Autodesk Inventor part; units mm, degrees
(part 11 of 12)
  line L8976 (-20.439, 26.0176) -> (-20.439, 27.0176)
  line L8977 (-20.439, 27.0176) -> (-19.439, 27.0176)
  line L8978 (-19.439, 27.0176) -> (-19.439, 26.0176)
  line L8979 (-20.4042, 26.0176) -> (-21.4042, 26.0176)
  line L8980 (-21.4042, 26.0176) -> (-21.4042, 27.0176)
  line L8981 (-21.4042, 27.0176) -> (-20.4042, 27.0176)
  line L8982 (-20.4042, 27.0176) -> (-20.4042, 26.0176)
  line L8983 (-21.0011, 26.0176) -> (-22.0011, 26.0176)
  line L8984 (-22.0011, 26.0176) -> (-22.0011, 27.0176)
  line L8985 (-22.0011, 27.0176) -> (-21.0011, 27.0176)
  line L8986 (-21.0011, 27.0176) -> (-21.0011, 26.0176)
  line L8987 (-22.1187, 26.0176) -> (-23.1187, 26.0176)
  line L8988 (-23.1187, 26.0176) -> (-23.1187, 27.0176)
  line L8989 (-23.1187, 27.0176) -> (-22.1187, 27.0176)
  line L8990 (-22.1187, 27.0176) -> (-22.1187, 26.0176)
  line L8991 (-12.9747, 26.043) -> (-13.9747, 26.043)
  line L8992 (-13.9747, 26.043) -> (-13.9747, 27.043)
  line L8993 (-13.9747, 27.043) -> (-12.9747, 27.043)
  line L8994 (-12.9747, 27.043) -> (-12.9747, 26.043)
  line L8995 (-14.5415, 26.5303) -> (-14.5669, 26.5303)
  line L8996 (-14.5669, 26.5303) -> (-14.5669, 26.5557)
  line L8997 (-14.5669, 26.5557) -> (-14.5415, 26.5557)
  line L8998 (-14.5415, 26.5557) -> (-14.5415, 26.5303)
  line L8999 (-14.6257, 26.043) -> (-15.6257, 26.043)
  line L9000 (-15.6257, 26.043) -> (-15.6257, 27.043)
  line L9001 (-15.6257, 27.043) -> (-14.6257, 27.043)
  line L9002 (-14.6257, 27.043) -> (-14.6257, 26.043)
  line L9003 (-19.439, 26.043) -> (-20.439, 26.043)
  line L9004 (-20.439, 26.043) -> (-20.439, 27.043)
  line L9005 (-20.439, 27.043) -> (-19.439, 27.043)
  line L9006 (-19.439, 27.043) -> (-19.439, 26.043)
  line L9007 (-20.4169, 26.043) -> (-21.4169, 26.043)
  line L9008 (-21.4169, 26.043) -> (-21.4169, 27.043)
  line L9009 (-21.4169, 27.043) -> (-20.4169, 27.043)
  line L9010 (-20.4169, 27.043) -> (-20.4169, 26.043)
  line L9011 (-21.0011, 26.043) -> (-22.0011, 26.043)
  line L9012 (-22.0011, 26.043) -> (-22.0011, 27.043)
  line L9013 (-22.0011, 27.043) -> (-21.0011, 27.043)
  line L9014 (-21.0011, 27.043) -> (-21.0011, 26.043)
  line L9015 (-22.1314, 26.043) -> (-23.1314, 26.043)
  line L9016 (-23.1314, 26.043) -> (-23.1314, 27.043)
  line L9017 (-23.1314, 27.043) -> (-22.1314, 27.043)
  line L9018 (-22.1314, 27.043) -> (-22.1314, 26.043)
  line L9019 (-13.0128, 26.0684) -> (-14.0128, 26.0684)
  line L9020 (-14.0128, 26.0684) -> (-14.0128, 27.0684)
  line L9021 (-14.0128, 27.0684) -> (-13.0128, 27.0684)
  line L9022 (-13.0128, 27.0684) -> (-13.0128, 26.0684)
  line L9023 (-14.0415, 26.0684) -> (-15.0415, 26.0684)
  line L9024 (-15.0415, 26.0684) -> (-15.0415, 27.0684)
  line L9025 (-15.0415, 27.0684) -> (-14.0415, 27.0684)
  line L9026 (-14.0415, 27.0684) -> (-14.0415, 26.0684)
  line L9027 (-14.6257, 26.0684) -> (-15.6257, 26.0684)
  line L9028 (-15.6257, 26.0684) -> (-15.6257, 27.0684)
  line L9029 (-15.6257, 27.0684) -> (-14.6257, 27.0684)
  line L9030 (-14.6257, 27.0684) -> (-14.6257, 26.0684)
  line L9031 (-13.0382, 26.0938) -> (-14.0382, 26.0938)
  line L9032 (-14.0382, 26.0938) -> (-14.0382, 27.0938)
  line L9033 (-14.0382, 27.0938) -> (-13.0382, 27.0938)
  line L9034 (-13.0382, 27.0938) -> (-13.0382, 26.0938)
  line L9035 (-14.0161, 26.0938) -> (-15.0161, 26.0938)
  line L9036 (-15.0161, 26.0938) -> (-15.0161, 27.0938)
  line L9037 (-15.0161, 27.0938) -> (-14.0161, 27.0938)
  line L9038 (-14.0161, 27.0938) -> (-14.0161, 26.0938)
  line L9039 (-14.613, 26.0938) -> (-15.613, 26.0938)
  line L9040 (-15.613, 26.0938) -> (-15.613, 27.0938)
  line L9041 (-15.613, 27.0938) -> (-14.613, 27.0938)
  line L9042 (-14.613, 27.0938) -> (-14.613, 26.0938)
  line L9043 (-13.0382, 26.1192) -> (-14.0382, 26.1192)
  line L9044 (-14.0382, 26.1192) -> (-14.0382, 27.1192)
  line L9045 (-14.0382, 27.1192) -> (-13.0382, 27.1192)
  line L9046 (-13.0382, 27.1192) -> (-13.0382, 26.1192)
  line L9047 (-13.9907, 26.1192) -> (-14.9907, 26.1192)
  line L9048 (-14.9907, 26.1192) -> (-14.9907, 27.1192)
  line L9049 (-14.9907, 27.1192) -> (-13.9907, 27.1192)
  line L9050 (-13.9907, 27.1192) -> (-13.9907, 26.1192)
  line L9051 (-14.613, 26.1192) -> (-15.613, 26.1192)
  line L9052 (-15.613, 26.1192) -> (-15.613, 27.1192)
  line L9053 (-15.613, 27.1192) -> (-14.613, 27.1192)
  line L9054 (-14.613, 27.1192) -> (-14.613, 26.1192)
  line L9055 (-13.0255, 26.1446) -> (-14.0255, 26.1446)
  line L9056 (-14.0255, 26.1446) -> (-14.0255, 27.1446)
  line L9057 (-14.0255, 27.1446) -> (-13.0255, 27.1446)
  line L9058 (-13.0255, 27.1446) -> (-13.0255, 26.1446)
  line L9059 (-13.9653, 26.1446) -> (-14.9653, 26.1446)
  line L9060 (-14.9653, 26.1446) -> (-14.9653, 27.1446)
  line L9061 (-14.9653, 27.1446) -> (-13.9653, 27.1446)
  line L9062 (-13.9653, 27.1446) -> (-13.9653, 26.1446)
  line L9063 (-14.613, 26.1446) -> (-15.613, 26.1446)
  line L9064 (-15.613, 26.1446) -> (-15.613, 27.1446)
  line L9065 (-15.613, 27.1446) -> (-14.613, 27.1446)
  line L9066 (-14.613, 27.1446) -> (-14.613, 26.1446)
  line L9067 (-13.0128, 26.17) -> (-14.0128, 26.17)
  line L9068 (-14.0128, 26.17) -> (-14.0128, 27.17)
  line L9069 (-14.0128, 27.17) -> (-13.0128, 27.17)
  line L9070 (-13.0128, 27.17) -> (-13.0128, 26.17)
  line L9071 (-13.9526, 26.17) -> (-14.9526, 26.17)
  line L9072 (-14.9526, 26.17) -> (-14.9526, 27.17)
  line L9073 (-14.9526, 27.17) -> (-13.9526, 27.17)
  line L9074 (-13.9526, 27.17) -> (-13.9526, 26.17)
  line L9075 (-14.6003, 26.17) -> (-15.6003, 26.17)
  line L9076 (-15.6003, 26.17) -> (-15.6003, 27.17)
  line L9077 (-15.6003, 27.17) -> (-14.6003, 27.17)
  line L9078 (-14.6003, 27.17) -> (-14.6003, 26.17)
  line L9079 (-13.0001, 26.1954) -> (-14.0001, 26.1954)
  line L9080 (-14.0001, 26.1954) -> (-14.0001, 27.1954)
  line L9081 (-14.0001, 27.1954) -> (-13.0001, 27.1954)
  line L9082 (-13.0001, 27.1954) -> (-13.0001, 26.1954)
  line L9083 (-13.9272, 26.1954) -> (-14.9272, 26.1954)
  line L9084 (-14.9272, 26.1954) -> (-14.9272, 27.1954)
  line L9085 (-14.9272, 27.1954) -> (-13.9272, 27.1954)
  line L9086 (-13.9272, 27.1954) -> (-13.9272, 26.1954)
  line L9087 (-14.6003, 26.1954) -> (-15.6003, 26.1954)
  line L9088 (-15.6003, 26.1954) -> (-15.6003, 27.1954)
  line L9089 (-15.6003, 27.1954) -> (-14.6003, 27.1954)
  line L9090 (-14.6003, 27.1954) -> (-14.6003, 26.1954)
  line L9091 (-12.9747, 26.2208) -> (-13.9747, 26.2208)
  line L9092 (-13.9747, 26.2208) -> (-13.9747, 27.2208)
  line L9093 (-13.9747, 27.2208) -> (-12.9747, 27.2208)
  line L9094 (-12.9747, 27.2208) -> (-12.9747, 26.2208)
  line L9095 (-13.9018, 26.2208) -> (-14.9018, 26.2208)
  line L9096 (-14.9018, 26.2208) -> (-14.9018, 27.2208)
  line L9097 (-14.9018, 27.2208) -> (-13.9018, 27.2208)
  line L9098 (-13.9018, 27.2208) -> (-13.9018, 26.2208)
  line L9099 (-14.5876, 26.2208) -> (-15.5876, 26.2208)
  line L9100 (-15.5876, 26.2208) -> (-15.5876, 27.2208)
  line L9101 (-15.5876, 27.2208) -> (-14.5876, 27.2208)
  line L9102 (-14.5876, 27.2208) -> (-14.5876, 26.2208)
  line L9103 (-12.9747, 26.2462) -> (-13.9747, 26.2462)
  line L9104 (-13.9747, 26.2462) -> (-13.9747, 27.2462)
  line L9105 (-13.9747, 27.2462) -> (-12.9747, 27.2462)
  line L9106 (-12.9747, 27.2462) -> (-12.9747, 26.2462)
  line L9107 (-13.8891, 26.2462) -> (-14.8891, 26.2462)
  line L9108 (-14.8891, 26.2462) -> (-14.8891, 27.2462)
  line L9109 (-14.8891, 27.2462) -> (-13.8891, 27.2462)
  line L9110 (-13.8891, 27.2462) -> (-13.8891, 26.2462)
  line L9111 (-14.5876, 26.2462) -> (-15.5876, 26.2462)
  line L9112 (-15.5876, 26.2462) -> (-15.5876, 27.2462)
  line L9113 (-15.5876, 27.2462) -> (-14.5876, 27.2462)
  line L9114 (-14.5876, 27.2462) -> (-14.5876, 26.2462)
  line L9115 (-12.9493, 26.2716) -> (-13.9493, 26.2716)
  line L9116 (-13.9493, 26.2716) -> (-13.9493, 27.2716)
  line L9117 (-13.9493, 27.2716) -> (-12.9493, 27.2716)
  line L9118 (-12.9493, 27.2716) -> (-12.9493, 26.2716)
  line L9119 (-13.8637, 26.2716) -> (-14.8637, 26.2716)
  line L9120 (-14.8637, 26.2716) -> (-14.8637, 27.2716)
  line L9121 (-14.8637, 27.2716) -> (-13.8637, 27.2716)
  line L9122 (-13.8637, 27.2716) -> (-13.8637, 26.2716)
  line L9123 (-14.5749, 26.2716) -> (-15.5749, 26.2716)
  line L9124 (-15.5749, 26.2716) -> (-15.5749, 27.2716)
  line L9125 (-15.5749, 27.2716) -> (-14.5749, 27.2716)
  line L9126 (-14.5749, 27.2716) -> (-14.5749, 26.2716)
  line L9127 (-12.9366, 26.297) -> (-13.9366, 26.297)
  line L9128 (-13.9366, 26.297) -> (-13.9366, 27.297)
  line L9129 (-13.9366, 27.297) -> (-12.9366, 27.297)
  line L9130 (-12.9366, 27.297) -> (-12.9366, 26.297)
  line L9131 (-13.8383, 26.297) -> (-14.8383, 26.297)
  line L9132 (-14.8383, 26.297) -> (-14.8383, 27.297)
  line L9133 (-14.8383, 27.297) -> (-13.8383, 27.297)
  line L9134 (-13.8383, 27.297) -> (-13.8383, 26.297)
  line L9135 (-14.5749, 26.297) -> (-15.5749, 26.297)
  line L9136 (-15.5749, 26.297) -> (-15.5749, 27.297)
  line L9137 (-15.5749, 27.297) -> (-14.5749, 27.297)
  line L9138 (-14.5749, 27.297) -> (-14.5749, 26.297)
  line L9139 (-12.9112, 26.3224) -> (-13.9112, 26.3224)
  line L9140 (-13.9112, 26.3224) -> (-13.9112, 27.3224)
  line L9141 (-13.9112, 27.3224) -> (-12.9112, 27.3224)
  line L9142 (-12.9112, 27.3224) -> (-12.9112, 26.3224)
  line L9143 (-13.8129, 26.3224) -> (-14.8129, 26.3224)
  line L9144 (-14.8129, 26.3224) -> (-14.8129, 27.3224)
  line L9145 (-14.8129, 27.3224) -> (-13.8129, 27.3224)
  line L9146 (-13.8129, 27.3224) -> (-13.8129, 26.3224)
  line L9147 (-14.5622, 26.3224) -> (-15.5622, 26.3224)
  line L9148 (-15.5622, 26.3224) -> (-15.5622, 27.3224)
  line L9149 (-15.5622, 27.3224) -> (-14.5622, 27.3224)
  line L9150 (-14.5622, 27.3224) -> (-14.5622, 26.3224)
  line L9151 (-12.9112, 26.3478) -> (-13.9112, 26.3478)
  line L9152 (-13.9112, 26.3478) -> (-13.9112, 27.3478)
  line L9153 (-13.9112, 27.3478) -> (-12.9112, 27.3478)
  line L9154 (-12.9112, 27.3478) -> (-12.9112, 26.3478)
  line L9155 (-13.8002, 26.3478) -> (-14.8002, 26.3478)
  line L9156 (-14.8002, 26.3478) -> (-14.8002, 27.3478)
  line L9157 (-14.8002, 27.3478) -> (-13.8002, 27.3478)
  line L9158 (-13.8002, 27.3478) -> (-13.8002, 26.3478)
  line L9159 (-14.5622, 26.3478) -> (-15.5622, 26.3478)
  line L9160 (-15.5622, 26.3478) -> (-15.5622, 27.3478)
  line L9161 (-15.5622, 27.3478) -> (-14.5622, 27.3478)
  line L9162 (-14.5622, 27.3478) -> (-14.5622, 26.3478)
  line L9163 (-12.8858, 26.3732) -> (-13.8858, 26.3732)
  line L9164 (-13.8858, 26.3732) -> (-13.8858, 27.3732)
  line L9165 (-13.8858, 27.3732) -> (-12.8858, 27.3732)
  line L9166 (-12.8858, 27.3732) -> (-12.8858, 26.3732)
  line L9167 (-13.7748, 26.3732) -> (-14.7748, 26.3732)
  line L9168 (-14.7748, 26.3732) -> (-14.7748, 27.3732)
  line L9169 (-14.7748, 27.3732) -> (-13.7748, 27.3732)
  line L9170 (-13.7748, 27.3732) -> (-13.7748, 26.3732)
  line L9171 (-14.5495, 26.3732) -> (-15.5495, 26.3732)
  line L9172 (-15.5495, 26.3732) -> (-15.5495, 27.3732)
  line L9173 (-15.5495, 27.3732) -> (-14.5495, 27.3732)
  line L9174 (-14.5495, 27.3732) -> (-14.5495, 26.3732)
  line L9175 (-12.8731, 26.3986) -> (-13.8731, 26.3986)
  line L9176 (-13.8731, 26.3986) -> (-13.8731, 27.3986)
  line L9177 (-13.8731, 27.3986) -> (-12.8731, 27.3986)
  line L9178 (-12.8731, 27.3986) -> (-12.8731, 26.3986)
  line L9179 (-13.7494, 26.3986) -> (-14.7494, 26.3986)
  line L9180 (-14.7494, 26.3986) -> (-14.7494, 27.3986)
  line L9181 (-14.7494, 27.3986) -> (-13.7494, 27.3986)
  line L9182 (-13.7494, 27.3986) -> (-13.7494, 26.3986)
  line L9183 (-14.5368, 26.3986) -> (-15.5368, 26.3986)
  line L9184 (-15.5368, 26.3986) -> (-15.5368, 27.3986)
  line L9185 (-15.5368, 27.3986) -> (-14.5368, 27.3986)
  line L9186 (-14.5368, 27.3986) -> (-14.5368, 26.3986)
  line L9187 (-12.8731, 26.424) -> (-13.8731, 26.424)
  line L9188 (-13.8731, 26.424) -> (-13.8731, 27.424)
  line L9189 (-13.8731, 27.424) -> (-12.8731, 27.424)
  line L9190 (-12.8731, 27.424) -> (-12.8731, 26.424)
  line L9191 (-13.724, 26.424) -> (-14.724, 26.424)
  line L9192 (-14.724, 26.424) -> (-14.724, 27.424)
  line L9193 (-14.724, 27.424) -> (-13.724, 27.424)
  line L9194 (-13.724, 27.424) -> (-13.724, 26.424)
  line L9195 (-14.5368, 26.424) -> (-15.5368, 26.424)
  line L9196 (-15.5368, 26.424) -> (-15.5368, 27.424)
  line L9197 (-15.5368, 27.424) -> (-14.5368, 27.424)
  line L9198 (-14.5368, 27.424) -> (-14.5368, 26.424)
  line L9199 (-12.8604, 26.4494) -> (-13.8604, 26.4494)
  line L9200 (-13.8604, 26.4494) -> (-13.8604, 27.4494)
  line L9201 (-13.8604, 27.4494) -> (-12.8604, 27.4494)
  line L9202 (-12.8604, 27.4494) -> (-12.8604, 26.4494)
  line L9203 (-13.7113, 26.4494) -> (-14.7113, 26.4494)
  line L9204 (-14.7113, 26.4494) -> (-14.7113, 27.4494)
  line L9205 (-14.7113, 27.4494) -> (-13.7113, 27.4494)
  line L9206 (-13.7113, 27.4494) -> (-13.7113, 26.4494)
  line L9207 (-14.5241, 26.4494) -> (-15.5241, 26.4494)
  line L9208 (-15.5241, 26.4494) -> (-15.5241, 27.4494)
  line L9209 (-15.5241, 27.4494) -> (-14.5241, 27.4494)
  line L9210 (-14.5241, 27.4494) -> (-14.5241, 26.4494)
  line L9211 (-12.835, 26.4748) -> (-13.835, 26.4748)
  line L9212 (-13.835, 26.4748) -> (-13.835, 27.4748)
  line L9213 (-13.835, 27.4748) -> (-12.835, 27.4748)
  line L9214 (-12.835, 27.4748) -> (-12.835, 26.4748)
  line L9215 (-13.6859, 26.4748) -> (-14.6859, 26.4748)
  line L9216 (-14.6859, 26.4748) -> (-14.6859, 27.4748)
  line L9217 (-14.6859, 27.4748) -> (-13.6859, 27.4748)
  line L9218 (-13.6859, 27.4748) -> (-13.6859, 26.4748)
  line L9219 (-14.5114, 26.4748) -> (-15.5114, 26.4748)
  line L9220 (-15.5114, 26.4748) -> (-15.5114, 27.4748)
  line L9221 (-15.5114, 27.4748) -> (-14.5114, 27.4748)
  line L9222 (-14.5114, 27.4748) -> (-14.5114, 26.4748)
  line L9223 (-12.8223, 26.5002) -> (-13.8223, 26.5002)
  line L9224 (-13.8223, 26.5002) -> (-13.8223, 27.5002)
  line L9225 (-13.8223, 27.5002) -> (-12.8223, 27.5002)
  line L9226 (-12.8223, 27.5002) -> (-12.8223, 26.5002)
  line L9227 (-13.6605, 26.5002) -> (-14.6605, 26.5002)
  line L9228 (-14.6605, 26.5002) -> (-14.6605, 27.5002)
  line L9229 (-14.6605, 27.5002) -> (-13.6605, 27.5002)
  line L9230 (-13.6605, 27.5002) -> (-13.6605, 26.5002)
  line L9231 (-14.4987, 26.5002) -> (-15.4987, 26.5002)
  line L9232 (-15.4987, 26.5002) -> (-15.4987, 27.5002)
  line L9233 (-15.4987, 27.5002) -> (-14.4987, 27.5002)
  line L9234 (-14.4987, 27.5002) -> (-14.4987, 26.5002)
  line L9235 (-12.8223, 26.5256) -> (-13.8223, 26.5256)
  line L9236 (-13.8223, 26.5256) -> (-13.8223, 27.5256)
  line L9237 (-13.8223, 27.5256) -> (-12.8223, 27.5256)
  line L9238 (-12.8223, 27.5256) -> (-12.8223, 26.5256)
  line L9239 (-13.6478, 26.5256) -> (-14.6478, 26.5256)
  line L9240 (-14.6478, 26.5256) -> (-14.6478, 27.5256)
  line L9241 (-14.6478, 27.5256) -> (-13.6478, 27.5256)
  line L9242 (-13.6478, 27.5256) -> (-13.6478, 26.5256)
  line L9243 (-14.486, 26.5256) -> (-15.486, 26.5256)
  line L9244 (-15.486, 26.5256) -> (-15.486, 27.5256)
  line L9245 (-15.486, 27.5256) -> (-14.486, 27.5256)
  line L9246 (-14.486, 27.5256) -> (-14.486, 26.5256)
  line L9247 (-13.2969, 27.0383) -> (-13.3223, 27.0383)
  line L9248 (-13.3223, 27.0383) -> (-13.3223, 27.0637)
  line L9249 (-13.3223, 27.0637) -> (-13.2969, 27.0637)
  line L9250 (-13.2969, 27.0637) -> (-13.2969, 27.0383)
  line L9251 (-13.6224, 26.551) -> (-14.6224, 26.551)
  line L9252 (-14.6224, 26.551) -> (-14.6224, 27.551)
  line L9253 (-14.6224, 27.551) -> (-13.6224, 27.551)
  line L9254 (-13.6224, 27.551) -> (-13.6224, 26.551)
  line L9255 (-14.4733, 26.551) -> (-15.4733, 26.551)
  line L9256 (-15.4733, 26.551) -> (-15.4733, 27.551)
  line L9257 (-15.4733, 27.551) -> (-14.4733, 27.551)
  line L9258 (-14.4733, 27.551) -> (-14.4733, 26.551)
  line L9259 (-13.597, 26.5764) -> (-14.597, 26.5764)
  line L9260 (-14.597, 26.5764) -> (-14.597, 27.5764)
  line L9261 (-14.597, 27.5764) -> (-13.597, 27.5764)
  line L9262 (-13.597, 27.5764) -> (-13.597, 26.5764)
  line L9263 (-14.4606, 26.5764) -> (-15.4606, 26.5764)
  line L9264 (-15.4606, 26.5764) -> (-15.4606, 27.5764)
  line L9265 (-15.4606, 27.5764) -> (-14.4606, 27.5764)
  line L9266 (-14.4606, 27.5764) -> (-14.4606, 26.5764)
  line L9267 (-13.5716, 26.6018) -> (-14.5716, 26.6018)
  line L9268 (-14.5716, 26.6018) -> (-14.5716, 27.6018)
  line L9269 (-14.5716, 27.6018) -> (-13.5716, 27.6018)
  line L9270 (-13.5716, 27.6018) -> (-13.5716, 26.6018)
  line L9271 (-14.4479, 26.6018) -> (-15.4479, 26.6018)
  line L9272 (-15.4479, 26.6018) -> (-15.4479, 27.6018)
  line L9273 (-15.4479, 27.6018) -> (-14.4479, 27.6018)
  line L9274 (-14.4479, 27.6018) -> (-14.4479, 26.6018)
  line L9275 (-13.5589, 26.6272) -> (-14.5589, 26.6272)
  line L9276 (-14.5589, 26.6272) -> (-14.5589, 27.6272)
  line L9277 (-14.5589, 27.6272) -> (-13.5589, 27.6272)
  line L9278 (-13.5589, 27.6272) -> (-13.5589, 26.6272)
  line L9279 (-14.4352, 26.6272) -> (-15.4352, 26.6272)
  line L9280 (-15.4352, 26.6272) -> (-15.4352, 27.6272)
  line L9281 (-15.4352, 27.6272) -> (-14.4352, 27.6272)
  line L9282 (-14.4352, 27.6272) -> (-14.4352, 26.6272)
  line L9283 (-13.5335, 26.6526) -> (-14.5335, 26.6526)
  line L9284 (-14.5335, 26.6526) -> (-14.5335, 27.6526)
  line L9285 (-14.5335, 27.6526) -> (-13.5335, 27.6526)
  line L9286 (-13.5335, 27.6526) -> (-13.5335, 26.6526)
  line L9287 (-14.4225, 26.6526) -> (-15.4225, 26.6526)
  line L9288 (-15.4225, 26.6526) -> (-15.4225, 27.6526)
  line L9289 (-15.4225, 27.6526) -> (-14.4225, 27.6526)
  line L9290 (-14.4225, 27.6526) -> (-14.4225, 26.6526)
  line L9291 (-13.5081, 26.678) -> (-14.5081, 26.678)
  line L9292 (-14.5081, 26.678) -> (-14.5081, 27.678)
  line L9293 (-14.5081, 27.678) -> (-13.5081, 27.678)
  line L9294 (-13.5081, 27.678) -> (-13.5081, 26.678)
  line L9295 (-14.4098, 26.678) -> (-15.4098, 26.678)
  line L9296 (-15.4098, 26.678) -> (-15.4098, 27.678)
  line L9297 (-15.4098, 27.678) -> (-14.4098, 27.678)
  line L9298 (-14.4098, 27.678) -> (-14.4098, 26.678)
  line L9299 (-13.5208, 26.7034) -> (-14.5208, 26.7034)
  line L9300 (-14.5208, 26.7034) -> (-14.5208, 27.7034)
  line L9301 (-14.5208, 27.7034) -> (-13.5208, 27.7034)
  line L9302 (-13.5208, 27.7034) -> (-13.5208, 26.7034)
  line L9303 (-14.3971, 26.7034) -> (-15.3971, 26.7034)
  line L9304 (-15.3971, 26.7034) -> (-15.3971, 27.7034)
  line L9305 (-15.3971, 27.7034) -> (-14.3971, 27.7034)
  line L9306 (-14.3971, 27.7034) -> (-14.3971, 26.7034)
  line L9307 (-13.5335, 26.7288) -> (-14.5335, 26.7288)
  line L9308 (-14.5335, 26.7288) -> (-14.5335, 27.7288)
  line L9309 (-14.5335, 27.7288) -> (-13.5335, 27.7288)
  line L9310 (-13.5335, 27.7288) -> (-13.5335, 26.7288)
  line L9311 (-14.3717, 26.7288) -> (-15.3717, 26.7288)
  line L9312 (-15.3717, 26.7288) -> (-15.3717, 27.7288)
  line L9313 (-15.3717, 27.7288) -> (-14.3717, 27.7288)
  line L9314 (-14.3717, 27.7288) -> (-14.3717, 26.7288)
  line L9315 (-13.5589, 26.7542) -> (-14.5589, 26.7542)
  line L9316 (-14.5589, 26.7542) -> (-14.5589, 27.7542)
  line L9317 (-14.5589, 27.7542) -> (-13.5589, 27.7542)
  line L9318 (-13.5589, 27.7542) -> (-13.5589, 26.7542)
  line L9319 (-14.359, 26.7542) -> (-15.359, 26.7542)
  line L9320 (-15.359, 26.7542) -> (-15.359, 27.7542)
  line L9321 (-15.359, 27.7542) -> (-14.359, 27.7542)
  line L9322 (-14.359, 27.7542) -> (-14.359, 26.7542)
  line L9323 (-13.5716, 26.7796) -> (-14.5716, 26.7796)
  line L9324 (-14.5716, 26.7796) -> (-14.5716, 27.7796)
  line L9325 (-14.5716, 27.7796) -> (-13.5716, 27.7796)
  line L9326 (-13.5716, 27.7796) -> (-13.5716, 26.7796)
  line L9327 (-14.3336, 26.7796) -> (-15.3336, 26.7796)
  line L9328 (-15.3336, 26.7796) -> (-15.3336, 27.7796)
  line L9329 (-15.3336, 27.7796) -> (-14.3336, 27.7796)
  line L9330 (-14.3336, 27.7796) -> (-14.3336, 26.7796)
  line L9331 (-13.597, 26.805) -> (-14.597, 26.805)
  line L9332 (-14.597, 26.805) -> (-14.597, 27.805)
  line L9333 (-14.597, 27.805) -> (-13.597, 27.805)
  line L9334 (-13.597, 27.805) -> (-13.597, 26.805)
  line L9335 (-14.3082, 26.805) -> (-15.3082, 26.805)
  line L9336 (-15.3082, 26.805) -> (-15.3082, 27.805)
  line L9337 (-15.3082, 27.805) -> (-14.3082, 27.805)
  line L9338 (-14.3082, 27.805) -> (-14.3082, 26.805)
  line L9339 (-13.6224, 26.8304) -> (-14.6224, 26.8304)
  line L9340 (-14.6224, 26.8304) -> (-14.6224, 27.8304)
  line L9341 (-14.6224, 27.8304) -> (-13.6224, 27.8304)
  line L9342 (-13.6224, 27.8304) -> (-13.6224, 26.8304)
  line L9343 (-14.2828, 26.8304) -> (-15.2828, 26.8304)
  line L9344 (-15.2828, 26.8304) -> (-15.2828, 27.8304)
  line L9345 (-15.2828, 27.8304) -> (-14.2828, 27.8304)
  line L9346 (-14.2828, 27.8304) -> (-14.2828, 26.8304)
  line L9347 (-13.6478, 26.8558) -> (-14.6478, 26.8558)
  line L9348 (-14.6478, 26.8558) -> (-14.6478, 27.8558)
  line L9349 (-14.6478, 27.8558) -> (-13.6478, 27.8558)
  line L9350 (-13.6478, 27.8558) -> (-13.6478, 26.8558)
  line L9351 (-14.7447, 27.3431) -> (-14.7701, 27.3431)
  line L9352 (-14.7701, 27.3431) -> (-14.7701, 27.3685)
  line L9353 (-14.7701, 27.3685) -> (-14.7447, 27.3685)
  line L9354 (-14.7447, 27.3685) -> (-14.7447, 27.3431)
  line L9355 (-13.6859, 26.8812) -> (-14.6859, 26.8812)
  line L9356 (-14.6859, 26.8812) -> (-14.6859, 27.8812)
  line L9357 (-14.6859, 27.8812) -> (-13.6859, 27.8812)
  line L9358 (-13.6859, 27.8812) -> (-13.6859, 26.8812)
  line L9359 (-13.724, 26.9066) -> (-14.724, 26.9066)
  line L9360 (-14.724, 26.9066) -> (-14.724, 27.9066)
  line L9361 (-14.724, 27.9066) -> (-13.724, 27.9066)
  line L9362 (-13.724, 27.9066) -> (-13.724, 26.9066)
  line L9363 (-13.7621, 26.932) -> (-14.7621, 26.932)
  line L9364 (-14.7621, 26.932) -> (-14.7621, 27.932)
  line L9365 (-14.7621, 27.932) -> (-13.7621, 27.932)
  line L9366 (-13.7621, 27.932) -> (-13.7621, 26.932)
  line L9367 (-13.7621, 26.9574) -> (-14.7621, 26.9574)
  line L9368 (-14.7621, 26.9574) -> (-14.7621, 27.9574)
  line L9369 (-14.7621, 27.9574) -> (-13.7621, 27.9574)
  line L9370 (-13.7621, 27.9574) -> (-13.7621, 26.9574)
  line L9371 (-9.56, 21.883) -> (-10.56, 21.883)
  line L9372 (-10.56, 21.883) -> (-10.56, 22.883)
  line L9373 (-10.56, 22.883) -> (-9.56, 22.883)
  line L9374 (-9.56, 22.883) -> (-9.56, 21.883)
  line L9375 (-9.56, 21.383) -> (-10.56, 21.383)
  line L9376 (-10.56, 21.383) -> (-10.56, 22.383)
  line L9377 (-10.56, 22.383) -> (-9.56, 22.383)
  line L9378 (-9.56, 22.383) -> (-9.56, 21.383)
  line L9379 (-9.56, 20.883) -> (-10.56, 20.883)
  line L9380 (-10.56, 20.883) -> (-10.56, 21.883)
  line L9381 (-10.56, 21.883) -> (-9.56, 21.883)
  line L9382 (-9.56, 21.883) -> (-9.56, 20.883)
  line L9383 (-9.56, 20.383) -> (-10.56, 20.383)
  line L9384 (-10.56, 20.383) -> (-10.56, 21.383)
  line L9385 (-10.56, 21.383) -> (-9.56, 21.383)
  line L9386 (-9.56, 21.383) -> (-9.56, 20.383)
  line L9387 (-9.56, 19.883) -> (-10.56, 19.883)
  line L9388 (-10.56, 19.883) -> (-10.56, 20.883)
  line L9389 (-10.56, 20.883) -> (-9.56, 20.883)
  line L9390 (-9.56, 20.883) -> (-9.56, 19.883)
  line L9391 (-9.56, 19.383) -> (-10.56, 19.383)
  line L9392 (-10.56, 19.383) -> (-10.56, 20.383)
  line L9393 (-10.56, 20.383) -> (-9.56, 20.383)
  line L9394 (-9.56, 20.383) -> (-9.56, 19.383)
  line L9395 (-9.56, 18.883) -> (-10.56, 18.883)
  line L9396 (-10.56, 18.883) -> (-10.56, 19.883)
  line L9397 (-10.56, 19.883) -> (-9.56, 19.883)
  line L9398 (-9.56, 19.883) -> (-9.56, 18.883)
  line L9399 (-9.56, 18.383) -> (-10.56, 18.383)
  line L9400 (-10.56, 18.383) -> (-10.56, 19.383)
  line L9401 (-10.56, 19.383) -> (-9.56, 19.383)
  line L9402 (-9.56, 19.383) -> (-9.56, 18.383)
  line L9403 (-9.56, 17.883) -> (-10.56, 17.883)
  line L9404 (-10.56, 17.883) -> (-10.56, 18.883)
  line L9405 (-10.56, 18.883) -> (-9.56, 18.883)
  line L9406 (-9.56, 18.883) -> (-9.56, 17.883)
  line L9407 (-9.56, 17.383) -> (-10.56, 17.383)
  line L9408 (-10.56, 17.383) -> (-10.56, 18.383)
  line L9409 (-10.56, 18.383) -> (-9.56, 18.383)
  line L9410 (-9.56, 18.383) -> (-9.56, 17.383)
  line L9411 (-9.56, 16.883) -> (-10.56, 16.883)
  line L9412 (-10.56, 16.883) -> (-10.56, 17.883)
  line L9413 (-10.56, 17.883) -> (-9.56, 17.883)
  line L9414 (-9.56, 17.883) -> (-9.56, 16.883)
  line L9415 (-9.56, 16.383) -> (-10.56, 16.383)
  line L9416 (-10.56, 16.383) -> (-10.56, 17.383)
  line L9417 (-10.56, 17.383) -> (-9.56, 17.383)
  line L9418 (-9.56, 17.383) -> (-9.56, 16.383)
  line L9419 (-9.56, 15.883) -> (-10.56, 15.883)
  line L9420 (-10.56, 15.883) -> (-10.56, 16.883)
  line L9421 (-10.56, 16.883) -> (-9.56, 16.883)
  line L9422 (-9.56, 16.883) -> (-9.56, 15.883)
  line L9423 (-9.56, 15.383) -> (-10.56, 15.383)
  line L9424 (-10.56, 15.383) -> (-10.56, 16.383)
  line L9425 (-10.56, 16.383) -> (-9.56, 16.383)
  line L9426 (-9.56, 16.383) -> (-9.56, 15.383)
  line L9427 (-9.56, 14.883) -> (-10.56, 14.883)
  line L9428 (-10.56, 14.883) -> (-10.56, 15.883)
  line L9429 (-10.56, 15.883) -> (-9.56, 15.883)
  line L9430 (-9.56, 15.883) -> (-9.56, 14.883)
  line L9431 (-9.56, 14.383) -> (-10.56, 14.383)
  line L9432 (-10.56, 14.383) -> (-10.56, 15.383)
  line L9433 (-10.56, 15.383) -> (-9.56, 15.383)
  line L9434 (-9.56, 15.383) -> (-9.56, 14.383)
  line L9435 (-9.56, 13.883) -> (-10.56, 13.883)
  line L9436 (-10.56, 13.883) -> (-10.56, 14.883)
  line L9437 (-10.56, 14.883) -> (-9.56, 14.883)
  line L9438 (-9.56, 14.883) -> (-9.56, 13.883)
  line L9439 (-9.56, 13.383) -> (-10.56, 13.383)
  line L9440 (-10.56, 13.383) -> (-10.56, 14.383)
  line L9441 (-10.56, 14.383) -> (-9.56, 14.383)
  line L9442 (-9.56, 14.383) -> (-9.56, 13.383)
  line L9443 (-9.56, 12.883) -> (-10.56, 12.883)
  line L9444 (-10.56, 12.883) -> (-10.56, 13.883)
  line L9445 (-10.56, 13.883) -> (-9.56, 13.883)
  line L9446 (-9.56, 13.883) -> (-9.56, 12.883)
  line L9447 (-9.56, 12.383) -> (-10.56, 12.383)
  line L9448 (-10.56, 12.383) -> (-10.56, 13.383)
  line L9449 (-10.56, 13.383) -> (-9.56, 13.383)
  line L9450 (-9.56, 13.383) -> (-9.56, 12.383)
  line L9451 (-9.56, 11.883) -> (-10.56, 11.883)
  line L9452 (-10.56, 11.883) -> (-10.56, 12.883)
  line L9453 (-10.56, 12.883) -> (-9.56, 12.883)
  line L9454 (-9.56, 12.883) -> (-9.56, 11.883)
  line L9455 (-9.56, 11.383) -> (-10.56, 11.383)
  line L9456 (-10.56, 11.383) -> (-10.56, 12.383)
  line L9457 (-10.56, 12.383) -> (-9.56, 12.383)
  line L9458 (-9.56, 12.383) -> (-9.56, 11.383)
  line L9459 (-9.56, 10.883) -> (-10.56, 10.883)
  line L9460 (-10.56, 10.883) -> (-10.56, 11.883)
  line L9461 (-10.56, 11.883) -> (-9.56, 11.883)
  line L9462 (-9.56, 11.883) -> (-9.56, 10.883)
  line L9463 (-9.56, 10.383) -> (-10.56, 10.383)
  line L9464 (-10.56, 10.383) -> (-10.56, 11.383)
  line L9465 (-10.56, 11.383) -> (-9.56, 11.383)
  line L9466 (-9.56, 11.383) -> (-9.56, 10.383)
  line L9467 (-9.56, 9.883) -> (-10.56, 9.883)
  line L9468 (-10.56, 9.883) -> (-10.56, 10.883)
  line L9469 (-10.56, 10.883) -> (-9.56, 10.883)
  line L9470 (-9.56, 10.883) -> (-9.56, 9.883)
  line L9471 (-11.28, 8.163) -> (-12.28, 8.163)
  line L9472 (-12.28, 8.163) -> (-12.28, 9.163)
  line L9473 (-12.28, 9.163) -> (-11.28, 9.163)
  line L9474 (-11.28, 9.163) -> (-11.28, 8.163)
  line L9475 (-11.78, 8.163) -> (-12.78, 8.163)
  line L9476 (-12.78, 8.163) -> (-12.78, 9.163)
  line L9477 (-12.78, 9.163) -> (-11.78, 9.163)
  line L9478 (-11.78, 9.163) -> (-11.78, 8.163)
  line L9479 (-12.28, 8.163) -> (-13.28, 8.163)
  line L9480 (-13.28, 8.163) -> (-13.28, 9.163)
  line L9481 (-13.28, 9.163) -> (-12.28, 9.163)
  line L9482 (-12.28, 9.163) -> (-12.28, 8.163)
  line L9483 (-12.78, 8.163) -> (-13.78, 8.163)
  line L9484 (-13.78, 8.163) -> (-13.78, 9.163)
  line L9485 (-13.78, 9.163) -> (-12.78, 9.163)
  line L9486 (-12.78, 9.163) -> (-12.78, 8.163)
  line L9487 (-13.28, 8.163) -> (-14.28, 8.163)
  line L9488 (-14.28, 8.163) -> (-14.28, 9.163)
  line L9489 (-14.28, 9.163) -> (-13.28, 9.163)
  line L9490 (-13.28, 9.163) -> (-13.28, 8.163)
  line L9491 (-13.78, 8.163) -> (-14.78, 8.163)
  line L9492 (-14.78, 8.163) -> (-14.78, 9.163)
  line L9493 (-14.78, 9.163) -> (-13.78, 9.163)
  line L9494 (-13.78, 9.163) -> (-13.78, 8.163)
  line L9495 (-14.28, 8.163) -> (-15.28, 8.163)
  line L9496 (-15.28, 8.163) -> (-15.28, 9.163)
  line L9497 (-15.28, 9.163) -> (-14.28, 9.163)
  line L9498 (-14.28, 9.163) -> (-14.28, 8.163)
  line L9499 (-14.78, 8.163) -> (-15.78, 8.163)
  line L9500 (-15.78, 8.163) -> (-15.78, 9.163)
  line L9501 (-15.78, 9.163) -> (-14.78, 9.163)
  line L9502 (-14.78, 9.163) -> (-14.78, 8.163)
  line L9503 (-15.28, 8.163) -> (-16.28, 8.163)
  line L9504 (-16.28, 8.163) -> (-16.28, 9.163)
  line L9505 (-16.28, 9.163) -> (-15.28, 9.163)
  line L9506 (-15.28, 9.163) -> (-15.28, 8.163)
  line L9507 (-15.78, 8.163) -> (-16.78, 8.163)
  line L9508 (-16.78, 8.163) -> (-16.78, 9.163)
  line L9509 (-16.78, 9.163) -> (-15.78, 9.163)
  line L9510 (-15.78, 9.163) -> (-15.78, 8.163)
  line L9511 (-16.28, 8.163) -> (-17.28, 8.163)
  line L9512 (-17.28, 8.163) -> (-17.28, 9.163)
  line L9513 (-17.28, 9.163) -> (-16.28, 9.163)
  line L9514 (-16.28, 9.163) -> (-16.28, 8.163)
  line L9515 (-16.78, 8.163) -> (-17.78, 8.163)
  line L9516 (-17.78, 8.163) -> (-17.78, 9.163)
  line L9517 (-17.78, 9.163) -> (-16.78, 9.163)
  line L9518 (-16.78, 9.163) -> (-16.78, 8.163)
  line L9519 (-17.28, 8.163) -> (-18.28, 8.163)
  line L9520 (-18.28, 8.163) -> (-18.28, 9.163)
  line L9521 (-18.28, 9.163) -> (-17.28, 9.163)
  line L9522 (-17.28, 9.163) -> (-17.28, 8.163)
  line L9523 (-17.78, 8.163) -> (-18.78, 8.163)
  line L9524 (-18.78, 8.163) -> (-18.78, 9.163)
  line L9525 (-18.78, 9.163) -> (-17.78, 9.163)
  line L9526 (-17.78, 9.163) -> (-17.78, 8.163)
  line L9527 (-18.28, 8.163) -> (-19.28, 8.163)
  line L9528 (-19.28, 8.163) -> (-19.28, 9.163)
  line L9529 (-19.28, 9.163) -> (-18.28, 9.163)
  line L9530 (-18.28, 9.163) -> (-18.28, 8.163)
  line L9531 (-18.78, 8.163) -> (-19.78, 8.163)
  line L9532 (-19.78, 8.163) -> (-19.78, 9.163)
  line L9533 (-19.78, 9.163) -> (-18.78, 9.163)
  line L9534 (-18.78, 9.163) -> (-18.78, 8.163)
  line L9535 (-19.28, 8.163) -> (-20.28, 8.163)
  line L9536 (-20.28, 8.163) -> (-20.28, 9.163)
  line L9537 (-20.28, 9.163) -> (-19.28, 9.163)
  line L9538 (-19.28, 9.163) -> (-19.28, 8.163)
  line L9539 (-19.78, 8.163) -> (-20.78, 8.163)
  line L9540 (-20.78, 8.163) -> (-20.78, 9.163)
  line L9541 (-20.78, 9.163) -> (-19.78, 9.163)
  line L9542 (-19.78, 9.163) -> (-19.78, 8.163)
  line L9543 (-20.28, 8.163) -> (-21.28, 8.163)
  line L9544 (-21.28, 8.163) -> (-21.28, 9.163)
  line L9545 (-21.28, 9.163) -> (-20.28, 9.163)
  line L9546 (-20.28, 9.163) -> (-20.28, 8.163)
  line L9547 (-20.78, 8.163) -> (-21.78, 8.163)
  line L9548 (-21.78, 8.163) -> (-21.78, 9.163)
  line L9549 (-21.78, 9.163) -> (-20.78, 9.163)
  line L9550 (-20.78, 9.163) -> (-20.78, 8.163)
  line L9551 (-21.28, 8.163) -> (-22.28, 8.163)
  line L9552 (-22.28, 8.163) -> (-22.28, 9.163)
  line L9553 (-22.28, 9.163) -> (-21.28, 9.163)
  line L9554 (-21.28, 9.163) -> (-21.28, 8.163)
  line L9555 (-21.78, 8.163) -> (-22.78, 8.163)
  line L9556 (-22.78, 8.163) -> (-22.78, 9.163)
  line L9557 (-22.78, 9.163) -> (-21.78, 9.163)
  line L9558 (-21.78, 9.163) -> (-21.78, 8.163)
  line L9559 (-22.28, 8.163) -> (-23.28, 8.163)
  line L9560 (-23.28, 8.163) -> (-23.28, 9.163)
  line L9561 (-23.28, 9.163) -> (-22.28, 9.163)
  line L9562 (-22.28, 9.163) -> (-22.28, 8.163)
  line L9563 (-22.78, 8.163) -> (-23.78, 8.163)
  line L9564 (-23.78, 8.163) -> (-23.78, 9.163)
  line L9565 (-23.78, 9.163) -> (-22.78, 9.163)
  line L9566 (-22.78, 9.163) -> (-22.78, 8.163)
  line L9567 (-23.28, 8.163) -> (-24.28, 8.163)
  line L9568 (-24.28, 8.163) -> (-24.28, 9.163)
  line L9569 (-24.28, 9.163) -> (-23.28, 9.163)
  line L9570 (-23.28, 9.163) -> (-23.28, 8.163)
  line L9571 (-25, 9.883) -> (-26, 9.883)
  line L9572 (-26, 9.883) -> (-26, 10.883)
  line L9573 (-26, 10.883) -> (-25, 10.883)
  line L9574 (-25, 10.883) -> (-25, 9.883)
  line L9575 (-25, 10.383) -> (-26, 10.383)
  line L9576 (-26, 10.383) -> (-26, 11.383)
  line L9577 (-26, 11.383) -> (-25, 11.383)
  line L9578 (-25, 11.383) -> (-25, 10.383)
  line L9579 (-25, 10.883) -> (-26, 10.883)
  line L9580 (-26, 10.883) -> (-26, 11.883)
  line L9581 (-26, 11.883) -> (-25, 11.883)
  line L9582 (-25, 11.883) -> (-25, 10.883)
  line L9583 (-25, 11.383) -> (-26, 11.383)
  line L9584 (-26, 11.383) -> (-26, 12.383)
  line L9585 (-26, 12.383) -> (-25, 12.383)
  line L9586 (-25, 12.383) -> (-25, 11.383)
  line L9587 (-25, 11.883) -> (-26, 11.883)
  line L9588 (-26, 11.883) -> (-26, 12.883)
  line L9589 (-26, 12.883) -> (-25, 12.883)
  line L9590 (-25, 12.883) -> (-25, 11.883)
  line L9591 (-25, 12.383) -> (-26, 12.383)
  line L9592 (-26, 12.383) -> (-26, 13.383)
  line L9593 (-26, 13.383) -> (-25, 13.383)
  line L9594 (-25, 13.383) -> (-25, 12.383)
  line L9595 (-25, 12.883) -> (-26, 12.883)
  line L9596 (-26, 12.883) -> (-26, 13.883)
  line L9597 (-26, 13.883) -> (-25, 13.883)
  line L9598 (-25, 13.883) -> (-25, 12.883)
  line L9599 (-25, 13.383) -> (-26, 13.383)
  line L9600 (-26, 13.383) -> (-26, 14.383)
  line L9601 (-26, 14.383) -> (-25, 14.383)
  line L9602 (-25, 14.383) -> (-25, 13.383)
  line L9603 (-25, 13.883) -> (-26, 13.883)
  line L9604 (-26, 13.883) -> (-26, 14.883)
  line L9605 (-26, 14.883) -> (-25, 14.883)
  line L9606 (-25, 14.883) -> (-25, 13.883)
  line L9607 (-25, 14.383) -> (-26, 14.383)
  line L9608 (-26, 14.383) -> (-26, 15.383)
  line L9609 (-26, 15.383) -> (-25, 15.383)
  line L9610 (-25, 15.383) -> (-25, 14.383)
  line L9611 (-25, 14.883) -> (-26, 14.883)
  line L9612 (-26, 14.883) -> (-26, 15.883)
  line L9613 (-26, 15.883) -> (-25, 15.883)
  line L9614 (-25, 15.883) -> (-25, 14.883)
  line L9615 (-25, 15.383) -> (-26, 15.383)
  line L9616 (-26, 15.383) -> (-26, 16.383)
  line L9617 (-26, 16.383) -> (-25, 16.383)
  line L9618 (-25, 16.383) -> (-25, 15.383)
  line L9619 (-25, 15.883) -> (-26, 15.883)
  line L9620 (-26, 15.883) -> (-26, 16.883)
  line L9621 (-26, 16.883) -> (-25, 16.883)
  line L9622 (-25, 16.883) -> (-25, 15.883)
  line L9623 (-25, 16.383) -> (-26, 16.383)
  line L9624 (-26, 16.383) -> (-26, 17.383)
  line L9625 (-26, 17.383) -> (-25, 17.383)
  line L9626 (-25, 17.383) -> (-25, 16.383)
  line L9627 (-25, 16.883) -> (-26, 16.883)
  line L9628 (-26, 16.883) -> (-26, 17.883)
  line L9629 (-26, 17.883) -> (-25, 17.883)
  line L9630 (-25, 17.883) -> (-25, 16.883)
  line L9631 (-25, 17.383) -> (-26, 17.383)
  line L9632 (-26, 17.383) -> (-26, 18.383)
  line L9633 (-26, 18.383) -> (-25, 18.383)
  line L9634 (-25, 18.383) -> (-25, 17.383)
  line L9635 (-25, 17.883) -> (-26, 17.883)
  line L9636 (-26, 17.883) -> (-26, 18.883)
  line L9637 (-26, 18.883) -> (-25, 18.883)
  line L9638 (-25, 18.883) -> (-25, 17.883)
  line L9639 (-25, 18.383) -> (-26, 18.383)
  line L9640 (-26, 18.383) -> (-26, 19.383)
  line L9641 (-26, 19.383) -> (-25, 19.383)
  line L9642 (-25, 19.383) -> (-25, 18.383)
  line L9643 (-25, 18.883) -> (-26, 18.883)
  line L9644 (-26, 18.883) -> (-26, 19.883)
  line L9645 (-26, 19.883) -> (-25, 19.883)
  line L9646 (-25, 19.883) -> (-25, 18.883)
  line L9647 (-25, 19.383) -> (-26, 19.383)
  line L9648 (-26, 19.383) -> (-26, 20.383)
  line L9649 (-26, 20.383) -> (-25, 20.383)
  line L9650 (-25, 20.383) -> (-25, 19.383)
  line L9651 (-25, 19.883) -> (-26, 19.883)
  line L9652 (-26, 19.883) -> (-26, 20.883)
  line L9653 (-26, 20.883) -> (-25, 20.883)
  line L9654 (-25, 20.883) -> (-25, 19.883)
  line L9655 (-25, 20.383) -> (-26, 20.383)
  line L9656 (-26, 20.383) -> (-26, 21.383)
  line L9657 (-26, 21.383) -> (-25, 21.383)
  line L9658 (-25, 21.383) -> (-25, 20.383)
  line L9659 (-25, 20.883) -> (-26, 20.883)
  line L9660 (-26, 20.883) -> (-26, 21.883)
  line L9661 (-26, 21.883) -> (-25, 21.883)
  line L9662 (-25, 21.883) -> (-25, 20.883)
  line L9663 (-25, 21.383) -> (-26, 21.383)
  line L9664 (-26, 21.383) -> (-26, 22.383)
  line L9665 (-26, 22.383) -> (-25, 22.383)
  line L9666 (-25, 22.383) -> (-25, 21.383)
  line L9667 (-25, 21.883) -> (-26, 21.883)
  line L9668 (-26, 21.883) -> (-26, 22.883)
  line L9669 (-26, 22.883) -> (-25, 22.883)
  line L9670 (-25, 22.883) -> (-25, 21.883)
  line L9671 (-23.28, 23.603) -> (-24.28, 23.603)
  line L9672 (-24.28, 23.603) -> (-24.28, 24.603)
  line L9673 (-24.28, 24.603) -> (-23.28, 24.603)
  line L9674 (-23.28, 24.603) -> (-23.28, 23.603)
  line L9675 (-22.78, 23.603) -> (-23.78, 23.603)
  line L9676 (-23.78, 23.603) -> (-23.78, 24.603)
  line L9677 (-23.78, 24.603) -> (-22.78, 24.603)
  line L9678 (-22.78, 24.603) -> (-22.78, 23.603)
  line L9679 (-22.28, 23.603) -> (-23.28, 23.603)
  line L9680 (-23.28, 23.603) -> (-23.28, 24.603)
  line L9681 (-23.28, 24.603) -> (-22.28, 24.603)
  line L9682 (-22.28, 24.603) -> (-22.28, 23.603)
  line L9683 (-21.78, 23.603) -> (-22.78, 23.603)
  line L9684 (-22.78, 23.603) -> (-22.78, 24.603)
  line L9685 (-22.78, 24.603) -> (-21.78, 24.603)
  line L9686 (-21.78, 24.603) -> (-21.78, 23.603)
  line L9687 (-21.28, 23.603) -> (-22.28, 23.603)
  line L9688 (-22.28, 23.603) -> (-22.28, 24.603)
  line L9689 (-22.28, 24.603) -> (-21.28, 24.603)
  line L9690 (-21.28, 24.603) -> (-21.28, 23.603)
  line L9691 (-20.78, 23.603) -> (-21.78, 23.603)
  line L9692 (-21.78, 23.603) -> (-21.78, 24.603)
  line L9693 (-21.78, 24.603) -> (-20.78, 24.603)
  line L9694 (-20.78, 24.603) -> (-20.78, 23.603)
  line L9695 (-20.28, 23.603) -> (-21.28, 23.603)
  line L9696 (-21.28, 23.603) -> (-21.28, 24.603)
  line L9697 (-21.28, 24.603) -> (-20.28, 24.603)
  line L9698 (-20.28, 24.603) -> (-20.28, 23.603)
  line L9699 (-19.78, 23.603) -> (-20.78, 23.603)
  line L9700 (-20.78, 23.603) -> (-20.78, 24.603)
  line L9701 (-20.78, 24.603) -> (-19.78, 24.603)
  line L9702 (-19.78, 24.603) -> (-19.78, 23.603)
  line L9703 (-19.28, 23.603) -> (-20.28, 23.603)
  line L9704 (-20.28, 23.603) -> (-20.28, 24.603)
  line L9705 (-20.28, 24.603) -> (-19.28, 24.603)
  line L9706 (-19.28, 24.603) -> (-19.28, 23.603)
  line L9707 (-18.78, 23.603) -> (-19.78, 23.603)
  line L9708 (-19.78, 23.603) -> (-19.78, 24.603)
  line L9709 (-19.78, 24.603) -> (-18.78, 24.603)
  line L9710 (-18.78, 24.603) -> (-18.78, 23.603)
  line L9711 (-18.28, 23.603) -> (-19.28, 23.603)
  line L9712 (-19.28, 23.603) -> (-19.28, 24.603)
  line L9713 (-19.28, 24.603) -> (-18.28, 24.603)
  line L9714 (-18.28, 24.603) -> (-18.28, 23.603)
  line L9715 (-17.78, 23.603) -> (-18.78, 23.603)
  line L9716 (-18.78, 23.603) -> (-18.78, 24.603)
  line L9717 (-18.78, 24.603) -> (-17.78, 24.603)
  line L9718 (-17.78, 24.603) -> (-17.78, 23.603)
  line L9719 (-17.28, 23.603) -> (-18.28, 23.603)
  line L9720 (-18.28, 23.603) -> (-18.28, 24.603)
  line L9721 (-18.28, 24.603) -> (-17.28, 24.603)
  line L9722 (-17.28, 24.603) -> (-17.28, 23.603)
  line L9723 (-16.78, 23.603) -> (-17.78, 23.603)
  line L9724 (-17.78, 23.603) -> (-17.78, 24.603)
  line L9725 (-17.78, 24.603) -> (-16.78, 24.603)
  line L9726 (-16.78, 24.603) -> (-16.78, 23.603)
  line L9727 (-16.28, 23.603) -> (-17.28, 23.603)
  line L9728 (-17.28, 23.603) -> (-17.28, 24.603)
  line L9729 (-17.28, 24.603) -> (-16.28, 24.603)
  line L9730 (-16.28, 24.603) -> (-16.28, 23.603)
  line L9731 (-15.78, 23.603) -> (-16.78, 23.603)
  line L9732 (-16.78, 23.603) -> (-16.78, 24.603)
  line L9733 (-16.78, 24.603) -> (-15.78, 24.603)
  line L9734 (-15.78, 24.603) -> (-15.78, 23.603)
  line L9735 (-15.28, 23.603) -> (-16.28, 23.603)
  line L9736 (-16.28, 23.603) -> (-16.28, 24.603)
  line L9737 (-16.28, 24.603) -> (-15.28, 24.603)
  line L9738 (-15.28, 24.603) -> (-15.28, 23.603)
  line L9739 (-14.78, 23.603) -> (-15.78, 23.603)
  line L9740 (-15.78, 23.603) -> (-15.78, 24.603)
  line L9741 (-15.78, 24.603) -> (-14.78, 24.603)
  line L9742 (-14.78, 24.603) -> (-14.78, 23.603)
  line L9743 (-14.28, 23.603) -> (-15.28, 23.603)
  line L9744 (-15.28, 23.603) -> (-15.28, 24.603)
  line L9745 (-15.28, 24.603) -> (-14.28, 24.603)
  line L9746 (-14.28, 24.603) -> (-14.28, 23.603)
  line L9747 (-13.78, 23.603) -> (-14.78, 23.603)
  line L9748 (-14.78, 23.603) -> (-14.78, 24.603)
  line L9749 (-14.78, 24.603) -> (-13.78, 24.603)
  line L9750 (-13.78, 24.603) -> (-13.78, 23.603)
  line L9751 (-13.28, 23.603) -> (-14.28, 23.603)
  line L9752 (-14.28, 23.603) -> (-14.28, 24.603)
  line L9753 (-14.28, 24.603) -> (-13.28, 24.603)
  line L9754 (-13.28, 24.603) -> (-13.28, 23.603)
  line L9755 (-12.78, 23.603) -> (-13.78, 23.603)
  line L9756 (-13.78, 23.603) -> (-13.78, 24.603)
  line L9757 (-13.78, 24.603) -> (-12.78, 24.603)
  line L9758 (-12.78, 24.603) -> (-12.78, 23.603)
  line L9759 (-12.28, 23.603) -> (-13.28, 23.603)
  line L9760 (-13.28, 23.603) -> (-13.28, 24.603)
  line L9761 (-13.28, 24.603) -> (-12.28, 24.603)
  line L9762 (-12.28, 24.603) -> (-12.28, 23.603)
  line L9763 (-11.78, 23.603) -> (-12.78, 23.603)
  line L9764 (-12.78, 23.603) -> (-12.78, 24.603)
  line L9765 (-12.78, 24.603) -> (-11.78, 24.603)
  line L9766 (-11.78, 24.603) -> (-11.78, 23.603)
  line L9767 (-11.28, 23.603) -> (-12.28, 23.603)
  line L9768 (-12.28, 23.603) -> (-12.28, 24.603)
  line L9769 (-12.28, 24.603) -> (-11.28, 24.603)
  line L9770 (-11.28, 24.603) -> (-11.28, 23.603)
  circle A493 centre (-19.9, 34.55) radius 0.17
  circle A494 centre (-19.1, 34.55) radius 0.17
  circle A495 centre (-18.3, 34.55) radius 0.17
  circle A496 centre (-17.5, 34.55) radius 0.17
  circle A497 centre (-16.7, 34.55) radius 0.17
  circle A498 centre (-15.9, 34.55) radius 0.17
  circle A499 centre (-19.9, 35.3) radius 0.17
  circle A500 centre (-19.1, 35.3) radius 0.17
  circle A501 centre (-18.3, 35.3) radius 0.17
  circle A502 centre (-17.5, 35.3) radius 0.17
  circle A503 centre (-16.7, 35.3) radius 0.17
  circle A504 centre (-15.9, 35.3) radius 0.17
  circle A505 centre (-19.9, 36.05) radius 0.17
  circle A506 centre (-15.9, 36.05) radius 0.17
  circle A507 centre (-19.9, 36.8) radius 0.17
  circle A508 centre (-15.9, 36.8) radius 0.17
  circle A509 centre (-19.9, 37.55) radius 0.17
  circle A510 centre (-19.1, 37.55) radius 0.17
  circle A511 centre (-18.3, 37.55) radius 0.17
  circle A512 centre (-17.5, 37.55) radius 0.17
  circle A513 centre (-16.7, 37.55) radius 0.17
  circle A514 centre (-15.9, 37.55) radius 0.17
  circle A515 centre (-19.9, 38.3) radius 0.17
  circle A516 centre (-19.1, 38.3) radius 0.17
  circle A517 centre (-18.3, 38.3) radius 0.17
  circle A518 centre (-17.5, 38.3) radius 0.17
  circle A519 centre (-16.7, 38.3) radius 0.17
  circle A520 centre (-15.9, 38.3) radius 0.17
  line L9771 (-8.103, 5.199) -> (-8.103, 4.199)
  line L9772 (-8.103, 4.199) -> (-9.103, 4.199)
  line L9773 (-9.103, 4.199) -> (-9.103, 5.199)
  line L9774 (-9.103, 5.199) -> (-8.103, 5.199)
  line L9775 (-8.103, 3.929) -> (-8.103, 2.929)
  line L9776 (-8.103, 2.929) -> (-9.103, 2.929)
  line L9777 (-9.103, 2.929) -> (-9.103, 3.929)
  line L9778 (-9.103, 3.929) -> (-8.103, 3.929)
  line L9779 (-8.103, 2.659) -> (-8.103, 1.659)
  line L9780 (-8.103, 1.659) -> (-9.103, 1.659)
  line L9781 (-9.103, 1.659) -> (-9.103, 2.659)
  line L9782 (-9.103, 2.659) -> (-8.103, 2.659)
  line L9783 (-8.103, 1.389) -> (-8.103, 0.389)
  line L9784 (-8.103, 0.389) -> (-9.103, 0.389)
  line L9785 (-9.103, 0.389) -> (-9.103, 1.389)
  line L9786 (-9.103, 1.389) -> (-8.103, 1.389)
  line L9787 (-13.503, 1.389) -> (-13.503, 0.389)
  line L9788 (-13.503, 0.389) -> (-14.503, 0.389)
  line L9789 (-14.503, 0.389) -> (-14.503, 1.389)
  line L9790 (-14.503, 1.389) -> (-13.503, 1.389)
  line L9791 (-13.503, 2.659) -> (-13.503, 1.659)
  line L9792 (-13.503, 1.659) -> (-14.503, 1.659)
  line L9793 (-14.503, 1.659) -> (-14.503, 2.659)
  line L9794 (-14.503, 2.659) -> (-13.503, 2.659)
  line L9795 (-13.503, 3.929) -> (-13.503, 2.929)
  line L9796 (-13.503, 2.929) -> (-14.503, 2.929)
  line L9797 (-14.503, 2.929) -> (-14.503, 3.929)
  line L9798 (-14.503, 3.929) -> (-13.503, 3.929)
  line L9799 (-13.503, 5.199) -> (-13.503, 4.199)
  line L9800 (-13.503, 4.199) -> (-14.503, 4.199)
  line L9801 (-14.503, 4.199) -> (-14.503, 5.199)
  line L9802 (-14.503, 5.199) -> (-13.503, 5.199)
  line L9803 (-10.803, 3.294) -> (-10.803, 2.294)
  line L9804 (-10.803, 2.294) -> (-11.803, 2.294)
  line L9805 (-11.803, 2.294) -> (-11.803, 3.294)
  line L9806 (-11.803, 3.294) -> (-10.803, 3.294)
  line L9807 (-31.641, 22.218) -> (-31.641, 21.068)
  line L9808 (-31.641, 21.068) -> (-32.791, 21.068)
  line L9809 (-32.791, 21.068) -> (-32.791, 22.218)
  line L9810 (-32.791, 22.218) -> (-31.641, 22.218)
  line L9811 (-34.266, 22.143) -> (-34.266, 21.143)
  line L9812 (-34.266, 21.143) -> (-35.266, 21.143)
  line L9813 (-35.266, 21.143) -> (-35.266, 22.143)
  line L9814 (-35.266, 22.143) -> (-34.266, 22.143)
  line L9815 (-32.166, 32.593) -> (-32.166, 31.593)
  line L9816 (-32.166, 31.593) -> (-33.166, 31.593)
  line L9817 (-33.166, 31.593) -> (-33.166, 32.593)
  line L9818 (-33.166, 32.593) -> (-32.166, 32.593)
  line L9819 (-33.366, 32.793) -> (-33.366, 31.793)
  line L9820 (-33.366, 31.793) -> (-34.366, 31.793)
  line L9821 (-34.366, 31.793) -> (-34.366, 32.793)
  line L9822 (-34.366, 32.793) -> (-33.366, 32.793)
  line L9823 (-34.416, 32.593) -> (-34.416, 31.593)
  line L9824 (-34.416, 31.593) -> (-35.416, 31.593)
  line L9825 (-35.416, 31.593) -> (-35.416, 32.593)
  line L9826 (-35.416, 32.593) -> (-34.416, 32.593)
  line L9827 (-30.666, 30.943) -> (-30.666, 29.943)
  line L9828 (-30.666, 29.943) -> (-31.666, 29.943)
  line L9829 (-31.666, 29.943) -> (-31.666, 30.943)
  line L9830 (-31.666, 30.943) -> (-30.666, 30.943)
  line L9831 (-30.666, 29.843) -> (-30.666, 28.843)
  line L9832 (-30.666, 28.843) -> (-31.666, 28.843)
  line L9833 (-31.666, 28.843) -> (-31.666, 29.843)
  line L9834 (-31.666, 29.843) -> (-30.666, 29.843)
  line L9835 (-30.666, 28.743) -> (-30.666, 27.743)
  line L9836 (-30.666, 27.743) -> (-31.666, 27.743)
  line L9837 (-31.666, 27.743) -> (-31.666, 28.743)
  line L9838 (-31.666, 28.743) -> (-30.666, 28.743)
  line L9839 (-30.666, 27.643) -> (-30.666, 26.643)
  line L9840 (-30.666, 26.643) -> (-31.666, 26.643)
  line L9841 (-31.666, 26.643) -> (-31.666, 27.643)
  line L9842 (-31.666, 27.643) -> (-30.666, 27.643)
  line L9843 (-30.666, 26.543) -> (-30.666, 25.543)
  line L9844 (-30.666, 25.543) -> (-31.666, 25.543)
  line L9845 (-31.666, 25.543) -> (-31.666, 26.543)
  line L9846 (-31.666, 26.543) -> (-30.666, 26.543)
  line L9847 (-30.666, 25.443) -> (-30.666, 24.443)
  line L9848 (-30.666, 24.443) -> (-31.666, 24.443)
  line L9849 (-31.666, 24.443) -> (-31.666, 25.443)
  line L9850 (-31.666, 25.443) -> (-30.666, 25.443)
  line L9851 (-30.666, 24.343) -> (-30.666, 23.343)
  line L9852 (-30.666, 23.343) -> (-31.666, 23.343)
  line L9853 (-31.666, 23.343) -> (-31.666, 24.343)
  line L9854 (-31.666, 24.343) -> (-30.666, 24.343)
  line L9855 (-30.666, 23.243) -> (-30.666, 22.243)
  line L9856 (-30.666, 22.243) -> (-31.666, 22.243)
  line L9857 (-31.666, 22.243) -> (-31.666, 23.243)
  line L9858 (-31.666, 23.243) -> (-30.666, 23.243)
  line L9859 (-25.87, 4.6275) -> (-24.87, 4.6275)
  line L9860 (-24.87, 4.6275) -> (-24.87, 3.6275)
  line L9861 (-24.87, 3.6275) -> (-25.87, 3.6275)
  line L9862 (-25.87, 3.6275) -> (-25.87, 4.6275)
  line L9863 (-26.52, 4.6275) -> (-25.52, 4.6275)
  line L9864 (-25.52, 4.6275) -> (-25.52, 3.6275)
  line L9865 (-25.52, 3.6275) -> (-26.52, 3.6275)
  line L9866 (-26.52, 3.6275) -> (-26.52, 4.6275)
  line L9867 (-27.17, 4.6275) -> (-26.17, 4.6275)
  line L9868 (-26.17, 4.6275) -> (-26.17, 3.6275)
  line L9869 (-26.17, 3.6275) -> (-27.17, 3.6275)
  line L9870 (-27.17, 3.6275) -> (-27.17, 4.6275)
  line L9871 (-27.82, 4.6275) -> (-26.82, 4.6275)
  line L9872 (-26.82, 4.6275) -> (-26.82, 3.6275)
  line L9873 (-26.82, 3.6275) -> (-27.82, 3.6275)
  line L9874 (-27.82, 3.6275) -> (-27.82, 4.6275)
  line L9875 (-28.47, 4.6275) -> (-27.47, 4.6275)
  line L9876 (-27.47, 4.6275) -> (-27.47, 3.6275)
  line L9877 (-27.47, 3.6275) -> (-28.47, 3.6275)
  line L9878 (-28.47, 3.6275) -> (-28.47, 4.6275)
  circle A521 centre (-23.37, 1.4525) radius 0.935
  circle A522 centre (-23.37, 1.4525) radius 0.935
  circle A523 centre (-23.37, 1.4525) radius 0.935
  circle A524 centre (-23.37, 1.4525) radius 0.935
  circle A525 centre (-29.97, 1.4525) radius 0.935
  circle A526 centre (-29.97, 1.4525) radius 0.935
  circle A527 centre (-29.97, 1.4525) radius 0.935
  circle A528 centre (-29.97, 1.4525) radius 0.935
  line L9879 (-23.97, 3.6275) -> (-23.97, 4.6275)
  line L9880 (-23.97, 4.6275) -> (-22.97, 4.6275)
  line L9881 (-22.97, 4.6275) -> (-22.97, 3.6275)
  line L9882 (-22.97, 3.6275) -> (-23.97, 3.6275)
  line L9883 (-30.37, 3.6275) -> (-30.37, 4.6275)
  line L9884 (-30.37, 4.6275) -> (-29.37, 4.6275)
  line L9885 (-29.37, 4.6275) -> (-29.37, 3.6275)
  line L9886 (-29.37, 3.6275) -> (-30.37, 3.6275)
  line L9887 (-24.52, 0.5025) -> (-26.42, 0.5025)
  line L9888 (-26.42, 0.5025) -> (-26.42, 2.4025)
  line L9889 (-26.42, 2.4025) -> (-24.52, 2.4025)
  line L9890 (-24.52, 2.4025) -> (-24.52, 0.5025)
  line L9891 (-26.92, 0.5025) -> (-28.82, 0.5025)
  line L9892 (-28.82, 0.5025) -> (-28.82, 2.4025)
  line L9893 (-28.82, 2.4025) -> (-26.92, 2.4025)
  line L9894 (-26.92, 2.4025) -> (-26.92, 0.5025)
  line L9895 (-4.669, 18.214) -> (-4.669, 17.214)
  line L9896 (-4.669, 17.214) -> (-5.669, 17.214)
  line L9897 (-5.669, 17.214) -> (-5.669, 18.214)
  line L9898 (-5.669, 18.214) -> (-4.669, 18.214)
  line L9899 (-4.669, 16.364) -> (-4.669, 15.364)
  line L9900 (-4.669, 15.364) -> (-5.669, 15.364)
  line L9901 (-5.669, 15.364) -> (-5.669, 16.364)
  line L9902 (-5.669, 16.364) -> (-4.669, 16.364)
  line L9903 (-6.219, 16.364) -> (-6.219, 15.364)
  line L9904 (-6.219, 15.364) -> (-7.219, 15.364)
  line L9905 (-7.219, 15.364) -> (-7.219, 16.364)
  line L9906 (-7.219, 16.364) -> (-6.219, 16.364)
  line L9907 (-6.219, 18.214) -> (-6.219, 17.214)
  line L9908 (-6.219, 17.214) -> (-7.219, 17.214)
  line L9909 (-7.219, 17.214) -> (-7.219, 18.214)
  line L9910 (-7.219, 18.214) -> (-6.219, 18.214)
  circle A529 centre (-29.591, 23.622) radius 0.2286
  circle A530 centre (-29.591, 23.622) radius 0.2286
  circle A531 centre (-32.385, 14.224) radius 0.2286